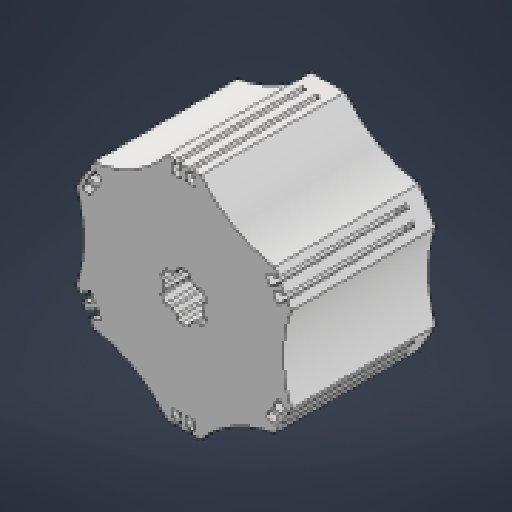
# Autodesk Inventor part: 3DPRINT,HUB
Saved by Autodesk Inventor 2026 (Build 300175000, 175)
## iProperties
Created: 2026-02-05
Part Number: 3DPRINT,HUB
Material: Generic
Document SubType Name: Modeling
Designer: Owen L
Density: 1 g/cm^3
Appearance: Default
Mass: 1846.51 g
Surface Area: 1357.43 cm^2
Volume: 1846.51 cm^3
Author: Owen L
Autodesk Inventor part; units mm, degrees
ref_plane "YZ Plane" through (0, 0, 0) normal (1, 0, 0) x (0, 1, 0)
ref_plane "XZ Plane" through (0, 0, 0) normal (0, 1, 0) x (-1, 0, 0)
ref_plane "XY Plane" through (0, 0, 0) normal (0, 0, 1) x (1, 0, 0)
sketch "Sketch1" plane through (0, 0, 0) normal (0, 0, 1) x (1, 0, 0)
  line L0 (0, 0) -> (0, 85.725) construction
  line L1 (-12.7, 85.725) -> (12.7, 85.725)
  line L2 (-80.59, 31.864) -> (-67.89, 53.861)
  line L3 (-67.89, -53.861) -> (-80.59, -31.864)
  line L4 (12.7, -85.725) -> (-12.7, -85.725)
  line L5 (80.59, -31.864) -> (67.89, -53.861)
  line L6 (67.89, 53.861) -> (80.59, 31.864)
  arc A0 (12.7, 85.725) -> (67.89, 53.861) centre (81.7917, 141.6674) ccw
  arc A1 (80.59, 31.864) -> (80.59, -31.864) centre (163.5834, 0) ccw
  arc A2 (67.89, -53.861) -> (12.7, -85.725) centre (81.7917, -141.6674) ccw
  arc A3 (-12.7, -85.725) -> (-67.89, -53.861) centre (-81.7917, -141.6674) ccw
  arc A4 (-80.59, -31.864) -> (-80.59, 31.864) centre (-163.5834, 0) ccw
  arc A5 (-67.89, 53.861) -> (-12.7, 85.725) centre (-81.7917, 141.6674) ccw
  dimension "d0" = 85.725
  dimension "d1" = 25.4
  dimension "d4" = 360
  dimension "d6" = 88.9
  constraints: 14 end point, 12 point on circle, 6 centre point, 5 equal radius, 1 horizontal, 1 midpoint, 1 vertical, 19 other
  measures "d0" distance of L0.start L0.end
  measures "d1" distance of L1.start L1.end
  measures "d6" radius of A0
extrude "Extrusion5" add sketch "Sketch1" along normal mid plane 82.55
sketch "Sketch7" plane through (0, 0, 41.275) normal (0, 0, 1) x (1, 0, 0)
  line L0 (-12.7, -85.725) -> (12.7, -85.725) projected
  line L1 (6.6675, -85.725) -> (6.6675, -82.55)
  line L2 (6.6675, -82.55) -> (8.5725, -82.55)
  line L3 (8.5725, -82.55) -> (8.5725, -76.2)
  line L4 (8.5725, -76.2) -> (1.5875, -76.2)
  line L5 (1.5875, -76.2) -> (1.5875, -82.55)
  line L6 (1.5875, -82.55) -> (3.4925, -82.55)
  line L7 (3.4925, -82.55) -> (3.4925, -85.725)
  line L8 (-3.4925, -85.725) -> (-3.4925, -82.55)
  line L9 (-3.4925, -82.55) -> (-1.5875, -82.55)
  line L10 (-1.5875, -82.55) -> (-1.5875, -76.2)
  line L11 (-1.5875, -76.2) -> (-8.5725, -76.2)
  line L12 (-8.5725, -76.2) -> (-8.5725, -82.55)
  line L13 (-8.5725, -82.55) -> (-6.6675, -82.55)
  line L14 (-6.6675, -82.55) -> (-6.6675, -85.725)
  line L15 (0, -85.725) -> (0, 0) construction
  dimension "d73" = 6.35
  dimension "d74" = 1.905
  dimension "d75" = 3.175
  dimension "d76" = 3.175
  dimension "d77" = 1.5875
  constraints: 30 end point, 10 perpendicular, 8 point on line, 6 equal length, 3 vertical, 1 midpoint, 1 other
  measures "d73" distance of L2.end L3.end
  measures "d74" distance of L1.end L2.end
  measures "d75" distance between parallel lines of L7 L1
  measures "d76" distance of L1.start L1.end
  measures "d77" distance between parallel lines of L15 L5
extrude "Extrusion6" cut sketch "Sketch7" against normal blind 76.2
pattern_circular "Circular Pattern3" count 6 over 360 about axis through (0, 0, -10) along (0, 0, 1) of "Extrusion6"
sketch "Sketch8" plane through (0, 0, 41.275) normal (0, 0, 1) x (1, 0, 0)
  arc A0 (13.8706, -10.5882) -> (16.1049, -6.7182) centre (0, 0) ccw projected
  arc A1 (11.1818, -11.0863) -> (13.8706, -10.5882) centre (12.251, -9.3519) ccw projected
  arc A2 (11.1818, -11.0863) -> (8.8244, -11.2207) centre (10.0994, -12.842) ccw projected
  arc A3 (5.3052, -13.2526) -> (8.8244, -11.2207) centre (0, 0) ccw projected
  arc A4 (5.3052, -13.2526) -> (4.0101, -15.2268) centre (6.0718, -15.1673) ccw projected
  arc A5 (2.2343, -17.3064) -> (4.0101, -15.2268) centre (1.9735, -15.2856) ccw projected
  arc A6 (-2.2343, -17.3064) -> (2.2343, -17.3064) centre (0, 0) ccw projected
  arc A7 (-4.0101, -15.2268) -> (-2.2343, -17.3064) centre (-1.9735, -15.2856) ccw projected
  arc A8 (-4.0101, -15.2268) -> (-5.3052, -13.2526) centre (-6.0718, -15.1673) ccw projected
  arc A9 (-8.8244, -11.2207) -> (-5.3052, -13.2526) centre (0, 0) ccw projected
  arc A10 (-8.8244, -11.2207) -> (-11.1818, -11.0863) centre (-10.0994, -12.842) ccw projected
  arc A11 (-13.8706, -10.5882) -> (-11.1818, -11.0863) centre (-12.251, -9.3519) ccw projected
  arc A12 (-16.1049, -6.7182) -> (-13.8706, -10.5882) centre (0, 0) ccw projected
  arc A13 (-15.1919, -4.1406) -> (-16.1049, -6.7182) centre (-14.2245, -5.9338) ccw projected
  arc A14 (-15.1919, -4.1406) -> (-14.1297, -2.0318) centre (-16.1712, -2.3254) ccw projected
  arc A15 (-14.1297, 2.0318) -> (-14.1297, -2.0318) centre (0, 0) ccw projected
  arc A16 (-14.1297, 2.0318) -> (-15.1919, 4.1406) centre (-16.1712, 2.3254) ccw projected
  arc A17 (-16.1049, 6.7182) -> (-15.1919, 4.1406) centre (-14.2245, 5.9338) ccw projected
  arc A18 (-13.8706, 10.5882) -> (-16.1049, 6.7182) centre (0, 0) ccw projected
  arc A19 (-11.1818, 11.0863) -> (-13.8706, 10.5882) centre (-12.251, 9.3519) ccw projected
  arc A20 (-11.1818, 11.0863) -> (-8.8244, 11.2207) centre (-10.0994, 12.842) ccw projected
  arc A21 (-5.3052, 13.2526) -> (-8.8244, 11.2207) centre (0, 0) ccw projected
  arc A22 (-5.3052, 13.2526) -> (-4.0101, 15.2268) centre (-6.0718, 15.1673) ccw projected
  arc A23 (-2.2343, 17.3064) -> (-4.0101, 15.2268) centre (-1.9735, 15.2856) ccw projected
  arc A24 (2.2343, 17.3064) -> (-2.2343, 17.3064) centre (0, 0) ccw projected
  arc A25 (4.0101, 15.2268) -> (2.2343, 17.3064) centre (1.9735, 15.2856) ccw projected
  arc A26 (4.0101, 15.2268) -> (5.3052, 13.2526) centre (6.0718, 15.1673) ccw projected
  arc A27 (8.8244, 11.2207) -> (5.3052, 13.2526) centre (0, 0) ccw projected
  arc A28 (8.8244, 11.2207) -> (11.1818, 11.0863) centre (10.0994, 12.842) ccw projected
  arc A29 (13.8706, 10.5882) -> (11.1818, 11.0863) centre (12.251, 9.3519) ccw projected
  arc A30 (16.1049, 6.7182) -> (13.8706, 10.5882) centre (0, 0) ccw projected
  arc A31 (15.1919, 4.1406) -> (16.1049, 6.7182) centre (14.2245, 5.9338) ccw projected
  arc A32 (15.1919, 4.1406) -> (14.1297, 2.0318) centre (16.1712, 2.3254) ccw projected
  arc A33 (14.1297, -2.0318) -> (14.1297, 2.0318) centre (0, 0) ccw projected
  arc A34 (14.1297, -2.0318) -> (15.1919, -4.1406) centre (16.1712, -2.3254) ccw projected
  arc A35 (16.1049, -6.7182) -> (15.1919, -4.1406) centre (14.2245, -5.9338) ccw projected
  arc A36 (12.0083, -9.7456) -> (12.6186, -9.6325) centre (12.251, -9.3519) ccw projected
  arc A37 (12.6186, -9.6325) -> (14.6513, -6.1118) centre (0, 0) ccw projected
  arc A38 (14.6513, -6.1118) -> (14.4441, -5.5267) centre (14.2245, -5.9338) ccw projected
  arc A39 (12.5707, -1.8076) -> (14.4441, -5.5267) centre (16.1712, -2.3254) ccw projected
  arc A40 (12.5707, -1.8076) -> (12.5707, 1.8076) centre (0, 0) ccw projected
  arc A41 (14.4441, 5.5267) -> (12.5707, 1.8076) centre (16.1712, 2.3254) ccw projected
  arc A42 (14.4441, 5.5267) -> (14.6513, 6.1118) centre (14.2245, 5.9338) ccw projected
  arc A43 (14.6513, 6.1118) -> (12.6186, 9.6325) centre (0, 0) ccw projected
  arc A44 (12.6186, 9.6325) -> (12.0083, 9.7456) centre (12.251, 9.3519) ccw projected
  arc A45 (7.8508, 9.9827) -> (12.0083, 9.7456) centre (10.0994, 12.842) ccw projected
  arc A46 (7.8508, 9.9827) -> (4.7199, 11.7904) centre (0, 0) ccw projected
  arc A47 (2.4358, 15.2723) -> (4.7199, 11.7904) centre (6.0718, 15.1673) ccw projected
  arc A48 (2.4358, 15.2723) -> (2.0327, 15.7443) centre (1.9735, 15.2856) ccw projected
  arc A49 (2.0327, 15.7443) -> (-2.0327, 15.7443) centre (0, 0) ccw projected
  arc A50 (-2.0327, 15.7443) -> (-2.4358, 15.2723) centre (-1.9735, 15.2856) ccw projected
  arc A51 (-4.7199, 11.7904) -> (-2.4358, 15.2723) centre (-6.0718, 15.1673) ccw projected
  arc A52 (-4.7199, 11.7904) -> (-7.8508, 9.9827) centre (0, 0) ccw projected
  arc A53 (-12.0083, 9.7456) -> (-7.8508, 9.9827) centre (-10.0994, 12.842) ccw projected
  arc A54 (-12.0083, 9.7456) -> (-12.6186, 9.6325) centre (-12.251, 9.3519) ccw projected
  arc A55 (-12.6186, 9.6325) -> (-14.6513, 6.1118) centre (0, 0) ccw projected
  arc A56 (-14.6513, 6.1118) -> (-14.4441, 5.5267) centre (-14.2245, 5.9338) ccw projected
  arc A57 (-12.5707, 1.8076) -> (-14.4441, 5.5267) centre (-16.1712, 2.3254) ccw projected
  arc A58 (-12.5707, 1.8076) -> (-12.5707, -1.8076) centre (0, 0) ccw projected
  arc A59 (-14.4441, -5.5267) -> (-12.5707, -1.8076) centre (-16.1712, -2.3254) ccw projected
  arc A60 (-14.4441, -5.5267) -> (-14.6513, -6.1118) centre (-14.2245, -5.9338) ccw projected
  arc A61 (-14.6513, -6.1118) -> (-12.6186, -9.6325) centre (0, 0) ccw projected
  arc A62 (-12.6186, -9.6325) -> (-12.0083, -9.7456) centre (-12.251, -9.3519) ccw projected
  arc A63 (-7.8508, -9.9827) -> (-12.0083, -9.7456) centre (-10.0994, -12.842) ccw projected
  arc A64 (-7.8508, -9.9827) -> (-4.7199, -11.7904) centre (0, 0) ccw projected
  arc A65 (-2.4358, -15.2723) -> (-4.7199, -11.7904) centre (-6.0718, -15.1673) ccw projected
  arc A66 (-2.4358, -15.2723) -> (-2.0327, -15.7443) centre (-1.9735, -15.2856) ccw projected
  arc A67 (-2.0327, -15.7443) -> (2.0327, -15.7443) centre (0, 0) ccw projected
  arc A68 (2.0327, -15.7443) -> (2.4358, -15.2723) centre (1.9735, -15.2856) ccw projected
  arc A69 (4.7199, -11.7904) -> (2.4358, -15.2723) centre (6.0718, -15.1673) ccw projected
  arc A70 (4.7199, -11.7904) -> (7.8508, -9.9827) centre (0, 0) ccw projected
  arc A71 (12.0083, -9.7456) -> (7.8508, -9.9827) centre (10.0994, -12.842) ccw projected
  arc A72 (16.3393, 6.816) -> (14.0725, 10.7423) centre (0, 0) ccw
  arc A73 (14.0725, 10.7423) -> (11.0485, 11.3025) centre (12.251, 9.3519) ccw
  arc A74 (8.9814, 11.4204) -> (11.0485, 11.3025) centre (10.0994, 12.842) ccw
  arc A75 (8.9814, 11.4204) -> (5.3996, 13.4884) centre (0, 0) ccw
  arc A76 (4.264, 15.2195) -> (5.3996, 13.4884) centre (6.0718, 15.1673) ccw
  arc A77 (4.264, 15.2195) -> (2.2669, 17.5583) centre (1.9735, 15.2856) ccw
  arc A78 (2.2669, 17.5583) -> (-2.2669, 17.5583) centre (0, 0) ccw
  arc A79 (-2.2669, 17.5583) -> (-4.264, 15.2195) centre (-1.9735, 15.2856) ccw
  arc A80 (-5.3996, 13.4884) -> (-4.264, 15.2195) centre (-6.0718, 15.1673) ccw
  arc A81 (-5.3996, 13.4884) -> (-8.9814, 11.4204) centre (0, 0) ccw
  arc A82 (-11.0485, 11.3025) -> (-8.9814, 11.4204) centre (-10.0994, 12.842) ccw
  arc A83 (-11.0485, 11.3025) -> (-14.0725, 10.7423) centre (-12.251, 9.3519) ccw
  arc A84 (-14.0725, 10.7423) -> (-16.3393, 6.816) centre (0, 0) ccw
  arc A85 (-16.3393, 6.816) -> (-15.3125, 3.917) centre (-14.2245, 5.9338) ccw
  arc A86 (-14.3811, 2.068) -> (-15.3125, 3.917) centre (-16.1712, 2.3254) ccw
  arc A87 (-14.3811, 2.068) -> (-14.3811, -2.068) centre (0, 0) ccw
  arc A88 (-15.3125, -3.917) -> (-14.3811, -2.068) centre (-16.1712, -2.3254) ccw
  arc A89 (-15.3125, -3.917) -> (-16.3393, -6.816) centre (-14.2245, -5.9338) ccw
  arc A90 (-16.3393, -6.816) -> (-14.0725, -10.7423) centre (0, 0) ccw
  arc A91 (-14.0725, -10.7423) -> (-11.0485, -11.3025) centre (-12.251, -9.3519) ccw
  arc A92 (-8.9814, -11.4204) -> (-11.0485, -11.3025) centre (-10.0994, -12.842) ccw
  arc A93 (-8.9814, -11.4204) -> (-5.3996, -13.4884) centre (0, 0) ccw
  arc A94 (-4.264, -15.2195) -> (-5.3996, -13.4884) centre (-6.0718, -15.1673) ccw
  arc A95 (-4.264, -15.2195) -> (-2.2669, -17.5583) centre (-1.9735, -15.2856) ccw
  arc A96 (-2.2669, -17.5583) -> (2.2669, -17.5583) centre (0, 0) ccw
  arc A97 (2.2669, -17.5583) -> (4.264, -15.2195) centre (1.9735, -15.2856) ccw
  arc A98 (5.3996, -13.4884) -> (4.264, -15.2195) centre (6.0718, -15.1673) ccw
  arc A99 (5.3996, -13.4884) -> (8.9814, -11.4204) centre (0, 0) ccw
  arc A100 (11.0485, -11.3025) -> (8.9814, -11.4204) centre (10.0994, -12.842) ccw
  arc A101 (11.0485, -11.3025) -> (14.0725, -10.7423) centre (12.251, -9.3519) ccw
  arc A102 (14.0725, -10.7423) -> (16.3393, -6.816) centre (0, 0) ccw
  arc A103 (16.3393, -6.816) -> (15.3125, -3.917) centre (14.2245, -5.9338) ccw
  arc A104 (14.3811, -2.068) -> (15.3125, -3.917) centre (16.1712, -2.3254) ccw
  arc A105 (14.3811, -2.068) -> (14.3811, 2.068) centre (0, 0) ccw
  arc A106 (15.3125, 3.917) -> (14.3811, 2.068) centre (16.1712, 2.3254) ccw
  arc A107 (15.3125, 3.917) -> (16.3393, 6.816) centre (14.2245, 5.9338) ccw
  point P0 (0, 0)
  dimension "d83" = 0.254
  constraints: 72 point on circle, 36 centre point, 35 other
  measures "d83" radial gap between concentric circles of A31 A107
extrude "Extrusion7" cut sketch "Sketch8" against normal through all contours A1 A2 A3 A4 A5 A6 A7 A8 A9 A10 A11 A12 A13 A14 A15 A16 A17 A18 A19 A20 A21 A22 A23 A24 A25 A26 A27 A28 A29 A30 A31 A32 A33 A34 A35 A0 | A71 A70 A69 A68 A67 A66 A65 A64 A63 A62 A61 A60 A59 A58 A57 A56 A55 A54 A53 A52 A51 A50 A49 A48 A47 A46 A45 A44 A43 A42 A41 A40 A39 A38 A37 A36 | A107 A106 A105 A104 A103 A102 A101 A100 A99 A98 A97 A96 A95 A94 A93 A92 A91 A90 A89 A88 A87 A86 A85 A84 A83 A82 A81 A80 A79 A78 A77 A76 A75 A74 A73 A72
fillet "Fillet3" radius 3.175 12 edges at (-80.59, 31.864, 0) (-67.89, 53.861, 0) (-12.7, 85.725, 0) (-80.59, -31.864, 0) (-67.89, -53.861, 0) (-12.7, -85.725, 0) (12.7, -85.725, 0) (67.89, -53.861, 0) (80.59, -31.864, 0) (67.89, 53.861, 0) (80.59, 31.864, 0) (12.7, 85.725, 0)
chamfer "Chamfer1" distance 1.5875 distance2 3.175 36 edges at (3.7161, -16.7737, -41.275) (4.5596, -14.1753, -41.275) (7.2645, -12.5825, -41.275) (9.9964, -11.0364, -41.275) (12.6684, -11.605, -41.275) (15.3321, -8.852, -41.275) (16.3845, -5.1686, -41.275) (14.556, -3.139, -41.275) (14.529, 0, -41.275) (14.556, 3.139, -41.275) (16.3845, 5.1686, -41.275) (15.3321, 8.852, -41.275) (12.6684, 11.605, -41.275) (9.9964, 11.0364, -41.275) (7.2645, 12.5825, -41.275) (4.5596, 14.1753, -41.275) (3.7161, 16.7737, -41.275) (0, 17.704, -41.275) (-3.7161, 16.7737, -41.275) (-4.5596, 14.1753, -41.275) (-7.2645, 12.5825, -41.275) (-9.9964, 11.0364, -41.275) (-12.6684, 11.605, -41.275) (-15.3321, 8.852, -41.275) (-16.3845, 5.1686, -41.275) (-14.556, 3.139, -41.275) (-14.529, 0, -41.275) (-14.556, -3.139, -41.275) (-16.3845, -5.1686, -41.275) (-15.3321, -8.852, -41.275) (-12.6684, -11.605, -41.275) (-9.9964, -11.0364, -41.275) (-7.2645, -12.5825, -41.275) (-4.5596, -14.1753, -41.275) (-3.7161, -16.7737, -41.275) (0, -17.704, -41.275) measured on face at (12.7595, 12.0967, -41.275) measured on face at (4.9777, 14.4496, -41.275) measured on face at (-7.5145, 13.0155, -41.275) measured on face at (-12.7595, 12.0967, -41.275) measured on face at (-4.9777, -14.4496, -41.275) measured on face at (16.8558, -5.0017, -41.275) measured on face at (7.5145, -13.0155, -41.275) measured on face at (-10.0249, -11.5356, -41.275) measured on face at (-7.5145, -13.0155, -41.275) measured on face at (0, -18.204, -41.275) measured on face at (-4.9777, 14.4496, -41.275) measured on face at (-15.7651, 9.102, -41.275) measured on face at (4.0963, -17.0984, -41.275) measured on face at (12.7595, -12.0967, -41.275) measured on face at (-16.8558, -5.0017, -41.275) measured on face at (-4.0963, 17.0984, -41.275) measured on face at (-15.029, 0, -41.275) measured on face at (4.0963, 17.0984, -41.275) measured on face at (-4.0963, -17.0984, -41.275) measured on face at (15.7651, 9.102, -41.275) measured on face at (-12.7595, -12.0967, -41.275) measured on face at (16.8558, 5.0017, -41.275) measured on face at (0, 18.204, -41.275) measured on face at (10.0249, -11.5356, -41.275) measured on face at (-15.7651, -9.102, -41.275) measured on face at (-10.0249, 11.5356, -41.275) measured on face at (-15.0026, 2.914, -41.275) measured on face at (4.9777, -14.4496, -41.275) measured on face at (15.029, 0, -41.275) measured on face at (-15.0026, -2.914, -41.275) measured on face at (-16.8558, 5.0017, -41.275) measured on face at (15.7651, -9.102, -41.275) measured on face at (15.0026, 2.914, -41.275) measured on face at (7.5145, 13.0155, -41.275) measured on face at (15.0026, -2.914, -41.275) measured on face at (10.0249, 11.5356, -41.275)
chamfer "Chamfer2" distance 1.5875 distance2 3.175 36 edges at (-3.7161, -16.7737, 41.275) (-4.5596, -14.1753, 41.275) (-7.2645, -12.5825, 41.275) (-9.9964, -11.0364, 41.275) (-12.6684, -11.605, 41.275) (-15.3321, -8.852, 41.275) (-16.3845, -5.1686, 41.275) (-14.556, -3.139, 41.275) (-14.529, 0, 41.275) (-14.556, 3.139, 41.275) (-16.3845, 5.1686, 41.275) (-15.3321, 8.852, 41.275) (-12.6684, 11.605, 41.275) (-9.9964, 11.0364, 41.275) (-7.2645, 12.5825, 41.275) (-4.5596, 14.1753, 41.275) (-3.7161, 16.7737, 41.275) (0, 17.704, 41.275) (3.7161, 16.7737, 41.275) (4.5596, 14.1753, 41.275) (7.2645, 12.5825, 41.275) (9.9964, 11.0364, 41.275) (12.6684, 11.605, 41.275) (15.3321, 8.852, 41.275) (16.3845, 5.1686, 41.275) (14.556, 3.139, 41.275) (14.529, 0, 41.275) (14.556, -3.139, 41.275) (16.3845, -5.1686, 41.275) (15.3321, -8.852, 41.275) (12.6684, -11.605, 41.275) (9.9964, -11.0364, 41.275) (7.2645, -12.5825, 41.275) (4.5596, -14.1753, 41.275) (3.7161, -16.7737, 41.275) (0, -17.704, 41.275) measured on face at (15.029, 0, 41.275) measured on face at (4.9777, -14.4496, 41.275) measured on face at (-15.0026, -2.914, 41.275) measured on face at (-16.8558, 5.0017, 41.275) measured on face at (15.0026, 2.914, 41.275) measured on face at (15.7651, -9.102, 41.275) measured on face at (10.0249, 11.5356, 41.275) measured on face at (7.5145, 13.0155, 41.275) measured on face at (15.0026, -2.914, 41.275) measured on face at (4.9777, 14.4496, 41.275) measured on face at (-7.5145, 13.0155, 41.275) measured on face at (-12.7595, 12.0967, 41.275) measured on face at (12.7595, 12.0967, 41.275) measured on face at (16.8558, -5.0017, 41.275) measured on face at (7.5145, -13.0155, 41.275) measured on face at (-4.9777, -14.4496, 41.275) measured on face at (-7.5145, -13.0155, 41.275) measured on face at (-10.0249, -11.5356, 41.275) measured on face at (0, -18.204, 41.275) measured on face at (-4.9777, 14.4496, 41.275) measured on face at (-15.7651, 9.102, 41.275) measured on face at (4.0963, -17.0984, 41.275) measured on face at (12.7595, -12.0967, 41.275) measured on face at (-16.8558, -5.0017, 41.275) measured on face at (-15.029, 0, 41.275) measured on face at (-4.0963, 17.0984, 41.275) measured on face at (4.0963, 17.0984, 41.275) measured on face at (-4.0963, -17.0984, 41.275) measured on face at (0, 18.204, 41.275) measured on face at (-12.7595, -12.0967, 41.275) measured on face at (15.7651, 9.102, 41.275) measured on face at (16.8558, 5.0017, 41.275) measured on face at (10.0249, -11.5356, 41.275) measured on face at (-15.7651, -9.102, 41.275) measured on face at (-15.0026, 2.914, 41.275) measured on face at (-10.0249, 11.5356, 41.275)
body "Solid3"
